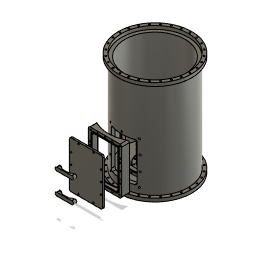
Smooth.SAQ.Pix.Vessel.5.10.2023. (Autodesk Fusion 360 design; units mm, degrees)
Autodesk Fusion 360 part; units mm, degrees
note: some values were not read from the file. Chosen so that the rebuilt part matches the saved one: which bodies a step acts on; which face or edge a step refers to. Set by a fixed rule: which sketch regions a step uses.
(part 1 of 2)
sketch "Vessel.Base" plane through (0, 0, 0) normal (0, 1, 0) x (1, 0, 0)
  circle A0 centre (0, 0) radius 40
  circle A1 centre (0, 0) radius 30
  circle A2 centre (0, 0) radius 100
  circle A3 centre (0, 0) radius 110
  line L0 (0, 0) -> (105, 0) construction
  circle A4 centre (105, 0) radius 2.3
  circle A5 centre (102.3674, 23.3647) radius 2.3
  circle A6 centre (94.6017, 45.5578) radius 2.3
  circle A7 centre (82.0923, 65.4664) radius 2.3
  circle A8 centre (65.4664, 82.0923) radius 2.3
  circle A9 centre (45.5578, 94.6017) radius 2.3
  circle A10 centre (23.3647, 102.3674) radius 2.3
  circle A11 centre (0, 105) radius 2.3
  circle A12 centre (-23.3647, 102.3674) radius 2.3
  circle A13 centre (-45.5578, 94.6017) radius 2.3
  circle A14 centre (-65.4664, 82.0923) radius 2.3
  circle A15 centre (-82.0923, 65.4664) radius 2.3
  circle A16 centre (-94.6017, 45.5578) radius 2.3
  circle A17 centre (-102.3674, 23.3647) radius 2.3
  circle A18 centre (-105, 0) radius 2.3
  circle A19 centre (-102.3674, -23.3647) radius 2.3
  circle A20 centre (-94.6017, -45.5578) radius 2.3
  circle A21 centre (-82.0923, -65.4664) radius 2.3
  circle A22 centre (-65.4664, -82.0923) radius 2.3
  circle A23 centre (-45.5578, -94.6017) radius 2.3
  circle A24 centre (-23.3647, -102.3674) radius 2.3
  circle A25 centre (0, -105) radius 2.3
  circle A26 centre (23.3647, -102.3674) radius 2.3
  circle A27 centre (45.5578, -94.6017) radius 2.3
  circle A28 centre (65.4664, -82.0923) radius 2.3
  circle A29 centre (82.0923, -65.4664) radius 2.3
  circle A30 centre (94.6017, -45.5578) radius 2.3
  circle A31 centre (102.3674, -23.3647) radius 2.3
  circle A32 centre (0, 0) radius 90
  circle A33 centre (0, 0) radius 50
  line L1 (0, 0) -> (45, 0) construction
  circle A34 centre (45, 0) radius 2.3
  circle A35 centre (40.5436, 19.5248) radius 2.3
  circle A36 centre (28.057, 35.1824) radius 2.3
  circle A37 centre (10.0134, 43.8718) radius 2.3
  circle A38 centre (-10.0134, 43.8718) radius 2.3
  circle A39 centre (-28.057, 35.1824) radius 2.3
  circle A40 centre (-40.5436, 19.5248) radius 2.3
  circle A41 centre (-45, 0) radius 2.3
  circle A42 centre (-40.5436, -19.5248) radius 2.3
  circle A43 centre (-28.057, -35.1824) radius 2.3
  circle A44 centre (-10.0134, -43.8718) radius 2.3
  circle A45 centre (10.0134, -43.8718) radius 2.3
  circle A46 centre (28.057, -35.1824) radius 2.3
  circle A47 centre (40.5436, -19.5248) radius 2.3
  circle A48 centre (0, 0) radius 35
  line L2 (0, 0) -> (0, -105) construction
  line L3 (0, 0) -> (0, -95) construction
  circle A49 centre (0, 0) radius 39
  circle A50 centre (0, 0) radius 49
  circle A51 centre (0, 0) radius 48
  circle A52 centre (0, 0) radius 32
  circle A53 centre (0, 0) radius 36 construction
  circle A54 centre (0, 0) radius 37
  circle A55 centre (0, 0) radius 38
  dimension "d1" = 80
  dimension "d2" = 60
  dimension "d3" = 200
  dimension "d4" = 220
  dimension "d5" = 4.6
  dimension "d7" = 360
  dimension "d10" = 180
  dimension "d85" = 100
  dimension "d105" = 45
  dimension "d106" = 4.6
  dimension "d108" = 360
  dimension "d111" = 70
  dimension "d187" = 105
  dimension "d188" = 95
  dimension "d324" = 78
  dimension "d325" = 98
  dimension "d326" = 96
  dimension "d349" = 64
  dimension "d524" = 72
  dimension "d525" = 74
  dimension "d526" = 76
  constraint coincident A0.centre A1.centre
  constraint concentric A1 A2
  constraint concentric A2 A3
  constraint horizontal L0
  constraint coincident L0.end A4.centre
  constraint concentric A0 A33
  constraint horizontal L1
  constraint coincident L1.end A34.centre
  constraint concentric A33 A48
  constraint vertical L2
  constraint parallel L2 L3
  constraint concentric A0 A50
  constraint concentric A48 A52
  constraint concentric A50 A53
  constraint concentric A33 A54
  constraint concentric A0 A55
  measures "d1" diameter of A0
  measures "d2" diameter of A1
  measures "d3" diameter of A2
  measures "d4" diameter of A3
  measures "d5" diameter of A4
  measures "d10" diameter of A32
  measures "d85" diameter of A33
  measures "d105" distance of A0.centre L1.end
  measures "d106" diameter of A34
  measures "d111" diameter of A48
  measures "d187" distance of A0.centre A25.centre
  measures "d188" distance of A0.centre L3.end
  measures "d324" diameter of A49
  measures "d325" diameter of A50
  measures "d326" diameter of A51
  measures "d349" diameter of A52
  measures "d524" diameter of A53
  measures "d525" diameter of A54
  measures "d526" diameter of A55
extrude "Extrude1" add sketch "Vessel.Base" along normal blind 10 contours A3 makes body 1
extrude "Extrude2" add sketch "Vessel.Base" along normal blind 300 separate body contours A2 makes body 2
extrude "Extrude3" add 1 faces at (-98.8073, 10, -35.1548) along direction (0, 1, 0) blind 10 separate body on bodies 1 makes body 3
move_body "Move1" bodies 3 to x (1, 0, 0) y (0, 1, 0) z (0, 0, 1) at (0, 280, 0)
extrude "Extrude5" add sketch "Vessel.Base" along normal blind 10 separate body contours A0 | A48 | A49 | A52 | A54 | A55 makes body 4
extrude "Extrude6" add sketch "Vessel.Base" along normal blind 11.6 contours A32 | A33 | A34 | A35 | A36 | A37 | A38 | A39 | A40 | A41 | A42 | A43 | A44 | A45 | A46 | A47 | A50 | A51 bodies 4
extrude "Extrude7" cut 1 faces at (36.4061, 10, 3.4777) along direction (0, -1, 0) blind 1.6 on bodies 4 bodies 4
sketch "Readout-Holder" plane through (0, 0, 0) normal (0, 1, 0) x (1, 0, 0)
  circle A0 centre (200, 0) radius 30
  circle A1 centre (200, 0) radius 1 construction
  circle A2 centre (210, 0) radius 1 construction
  circle A3 centre (220, 0) radius 1 construction
  circle A4 centre (180, 0) radius 1 construction
  circle A5 centre (205, 8.6603) radius 1 construction
  circle A6 centre (195, 8.6603) radius 1 construction
  circle A7 centre (190, 0) radius 1 construction
  circle A8 centre (195, -8.6603) radius 1 construction
  circle A9 centre (205, -8.6603) radius 1 construction
  circle A10 centre (210, 17.3205) radius 1 construction
  circle A11 centre (190, 17.3205) radius 1 construction
  circle A12 centre (180, 0) radius 1 construction
  circle A13 centre (190, -17.3205) radius 1 construction
  circle A14 centre (210, -17.3205) radius 1 construction
  circle A15 centre (200, 17.3205) radius 1 construction
  circle A16 centre (200, -17.3205) radius 1 construction
  circle A17 centre (185, 8.6603) radius 1 construction
  circle A18 centre (215, 8.6603) radius 1 construction
  circle A19 centre (185, -8.6603) radius 1 construction
  circle A20 centre (215, -8.6603) radius 1 construction
  circle A21 centre (200, 0) radius 40
  circle A22 centre (200, 0) radius 4.5
  circle A23 centre (210, 0) radius 4.5
  circle A24 centre (220, 0) radius 4.5
  circle A25 centre (215, 8.6603) radius 4.5
  circle A26 centre (205, 8.6603) radius 4.5
  circle A27 centre (195, 8.6603) radius 4.5
  circle A28 centre (185, 8.6603) radius 4.5
  circle A29 centre (190, 17.3205) radius 4.5
  circle A30 centre (200, 17.3205) radius 4.5
  circle A31 centre (210, 17.3205) radius 4.5
  circle A32 centre (190, 0) radius 4.5
  circle A33 centre (180, 0) radius 4.5
  circle A34 centre (185, -8.6603) radius 4.5
  circle A35 centre (195, -8.6603) radius 4.5
  circle A36 centre (205, -8.6603) radius 4.5
  circle A37 centre (215, -8.6603) radius 4.5
  circle A38 centre (190, -17.3205) radius 4.5
  circle A39 centre (200, -17.3205) radius 4.5
  circle A40 centre (210, -17.3205) radius 4.5
  circle A41 centre (200, 0) radius 50
  line L0 (200, 0) -> (245, 0) construction
  circle A42 centre (245, 0) radius 2.3
  circle A43 centre (240.5436, 19.5248) radius 2.3
  circle A44 centre (228.057, 35.1824) radius 2.3
  circle A45 centre (210.0134, 43.8718) radius 2.3
  circle A46 centre (189.9866, 43.8718) radius 2.3
  circle A47 centre (171.943, 35.1824) radius 2.3
  circle A48 centre (159.4564, 19.5248) radius 2.3
  circle A49 centre (159.4564, -19.5248) radius 2.3
  circle A50 centre (171.943, -35.1824) radius 2.3
  circle A51 centre (189.9866, -43.8718) radius 2.3
  circle A52 centre (210.0134, -43.8718) radius 2.3
  circle A53 centre (228.057, -35.1824) radius 2.3
  circle A54 centre (240.5436, -19.5248) radius 2.3
  line L1 (215, 8.6603) -> (225, 8.6603) construction
  circle A55 centre (225, 8.6603) radius 1 construction
  circle A56 centre (225, 8.6603) radius 4.5
  circle A57 centre (200, 0) radius 35 construction
  circle A58 centre (200, 0) radius 36.25
  circle A59 centre (200, 0) radius 38.75
  circle A60 centre (200, 0) radius 49
  circle A61 centre (200, 0) radius 34
  circle A62 centre (200, 0) radius 32 construction
  circle A63 centre (200, 0) radius 33
  line L2 (195, -8.6603) -> (185, -8.6603) construction
  line L3 (200, 0) -> (155, 0) construction
  circle A64 centre (155, 0) radius 2.3
  arc A65 (159.4515, 19.5147) -> (155, 0) centre (200, 0) ccw construction
  line L4 (200, 0) -> (159.4515, 19.5147) construction
  line L5 (200, 0) -> (155, 0) construction
  circle A66 centre (200, 0) radius 42
  line L6 (200, 0) -> (200, 35) construction
  circle A67 centre (200, 35) radius 3
  circle A68 centre (169.6891, -17.5) radius 3
  circle A69 centre (230.3109, -17.5) radius 3
  circle A70 centre (200, 32) radius 1
  line L7 (200, 0) -> (200, 32) construction
  circle A71 centre (172.2872, -16) radius 1
  circle A72 centre (227.7128, -16) radius 1
  dimension "d23" = 60
  dimension "d28" = 20
  dimension "d29" = 0
  dimension "d32" = -20
  dimension "d33" = 0
  dimension "d35" = 360
  dimension "d37" = 360
  dimension "d52" = 80
  dimension "d74" = 9
  dimension "d102" = 360
  dimension "d226" = 70
  dimension "d227" = 72.5
  dimension "d228" = 77.5
  dimension "d330" = 98
  dimension "d358" = 68
  dimension "d359" = 64
  dimension "d360" = 66
  dimension "d362" = 10
  dimension "d363" = 45
  dimension "d364" = 4.6
  dimension "d365" = 25.7
  dimension "d378" = 84
  dimension "d397" = 35
  dimension "d398" = 6
  dimension "d400" = 360
  dimension "d404" = 2
  dimension "d405" = 32
  dimension "d407" = 360
  constraint concentric A0 A1
  constraint concentric A0 A21
  constraint concentric A1 A22
  constraint concentric A2 A23
  constraint concentric A3 A24
  constraint concentric A18 A25
  constraint concentric A5 A26
  constraint concentric A6 A27
  constraint concentric A17 A28
  constraint concentric A11 A29
  constraint concentric A15 A30
  constraint concentric A10 A31
  constraint concentric A7 A32
  constraint concentric A12 A33
  constraint concentric A19 A34
  constraint concentric A8 A35
  constraint concentric A9 A36
  constraint concentric A20 A37
  constraint concentric A13 A38
  constraint concentric A16 A39
  constraint concentric A14 A40
  constraint concentric A22 A41
  constraint coincident A0.centre A1.centre
  constraint horizontal L0
  constraint coincident L0.end A42.centre
  constraint horizontal L1
  constraint coincident A18.centre A25.centre
  constraint coincident L1.end A55.centre
  constraint concentric A55 A56
  constraint concentric A41 A57
  constraint concentric A57 A58
  constraint concentric A58 A59
  constraint concentric A1 A60
  constraint concentric A0 A61
  constraint concentric A41 A62
  constraint concentric A0 A63
  constraint coincident A8.centre A35.centre
  constraint horizontal L2
  constraint horizontal L3
  constraint coincident L3.end A64.centre
  constraint concentric A21 A66
  constraint vertical L6
  constraint coincident L6.end A67.centre
  constraint coincident A67 A70.centre
  constraint coincident A62 A70.centre
  constraint parallel L6 L7
  measures "d23" diameter of A0
  measures "d52" diameter of A21
  measures "d74" diameter of A34
  measures "d226" diameter of A57
  measures "d227" diameter of A58
  measures "d228" diameter of A59
  measures "d330" diameter of A60
  measures "d358" diameter of A61
  measures "d359" diameter of A62
  measures "d360" diameter of A63
  measures "d362" distance of A8.centre A19.centre
  measures "d363" distance of A0.centre L3.end
  measures "d364" diameter of A64
  measures "d365" angle of L4 L5
  measures "d378" diameter of A66
  measures "d397" distance of A0.centre L6.end
  measures "d398" diameter of A67
  measures "d404" diameter of A70
  measures "d405" distance of A0.centre A70.centre
extrude "Extrude16" cut sketch "Vessel.Base" along normal blind 18 contours A1 bodies 4
extrude "Extrude17" cut sketch "Vessel.Base" along normal blind 14 contours A0 | A33 | A34 | A35 | A36 | A37 | A38 | A39 | A40 | A41 | A42 | A43 | A44 | A45 | A46 | A47 | A48 | A49 | A50 | A51 | A52 | A54 | A55 bodies 4
extrude "Extrude18" add sketch "Vessel.Base" along normal blind 2 contours A0 | A33 | A34 | A35 | A36 | A37 | A38 | A39 | A40 | A41 | A42 | A43 | A44 | A45 | A46 | A47 | A48 | A49 | A50 | A51 | A52 | A54 | A55 bodies 4
extrude "Extrude19" add 1 faces at (43.0355, 2, 3.9745) along direction (0, 1, 0) blind 4 on bodies 4 bodies 4
extrude "Extrude20" add sketch "Readout-Holder" along normal blind 8 separate body contours A0 A56 | A21 | A41 | A42 | A43 | A44 | A45 | A46 | A47 | A48 | A49 | A50 | A51 | A52 | A53 | A54 | A58 A61 A67 A69 | A58 A61 A67 | A58 A67 | A58 A69 | A58 A61 A69 | A58 A61 A67 A68 | A58 A61 A68 A69 | A61 A63 A67 A69 | A61 A63 A69 | A58 A61 A68 | A58 A68 | A61 A63 A67 A68 | A61 A63 A67 | A61 A63 A68 A69 | A63 A67 A68 A69 A70 A71 A72 | A63 A69 A72 | A61 A63 A68 | A63 A67 A70 | A63 A67 A70 | A63 A69 A72 | A69 A72 | A69 A72 | A63 A68 A71 | A67 A70 | A67 A70 | A63 A68 A71 | A68 A71 | A68 A71 | A59 | A60 | A64 | A66 picked at (228.6545, 9.8725) makes body 5
extrude "Extrude21" cut sketch "Readout-Holder" along normal blind 4 contours A0 A56 | A21 | A41 | A42 | A43 | A44 | A45 | A46 | A47 | A48 | A49 | A50 | A51 | A52 | A53 | A54 | A58 A61 A67 A69 | A58 A61 A67 | A58 A67 | A58 A69 | A58 A61 A69 | A58 A61 A67 A68 | A58 A61 A68 A69 | A61 A63 A67 A69 | A61 A63 A69 | A58 A61 A68 | A58 A68 | A61 A63 A67 A68 | A61 A63 A67 | A61 A63 A68 A69 | A63 A67 A68 A69 A70 A71 A72 | A63 A69 A72 | A61 A63 A68 | A63 A67 A70 | A63 A67 A70 | A63 A69 A72 | A69 A72 | A69 A72 | A63 A68 A71 | A67 A70 | A67 A70 | A63 A68 A71 | A68 A71 | A68 A71 | A59 | A60 | A64 | A66 picked at (228.6545, 9.8725) bodies 5
extrude "Extrude22" add sketch "Readout-Holder" along normal blind 8 contours A0 A56 | A0 A56 picked at (176.7568, 7.7937) picked at (225.7718, 9.0442) bodies 5
extrude "Extrude23" cut sketch "Readout-Holder" along normal blind 20 contours A42 | A43 | A44 | A45 | A46 | A47 | A48 | A49 | A50 | A51 | A52 | A53 | A54 bodies 5
extrude "Extrude24" cut sketch "Vessel.Base" along normal blind 24 contours A34 | A35 | A36 | A37 | A38 | A39 | A40 | A41 | A42 | A43 | A44 | A45 | A46 | A47 bodies 4
extrude "Extrude25" cut sketch "Vessel.Base" along normal blind 1 from surface at 5 contours A0 | A49 | A54 | A55 bodies 4
sketch "Door.Hole" plane through (0, 0, 0) normal (0, 0, 1) x (1, 0, 0)
  line L0 (-35, 30) -> (35, 30)
  line L1 (40, 35) -> (40, 145)
  line L2 (35, 150) -> (-35, 150)
  line L3 (-40, 145) -> (-40, 35)
  line L4 (-45, 20) -> (45, 20)
  line L5 (50, 25) -> (50, 155)
  line L6 (45, 160) -> (-45, 160)
  line L7 (-50, 155) -> (-50, 25)
  circle A0 centre (0, 155) radius 2.3
  circle A1 centre (45, 155) radius 2.3 construction
  circle A2 centre (-45, 111.6667) radius 2.3
  circle A3 centre (45, 111.6667) radius 2.3
  circle A4 centre (-45, 68.3333) radius 2.3
  circle A5 centre (45, 68.3333) radius 2.3
  circle A6 centre (0, 25) radius 2.3
  arc A7 (-35, 150) -> (-40, 145) centre (-35, 145) ccw
  arc A8 (40, 145) -> (35, 150) centre (35, 145) ccw
  arc A9 (-40, 35) -> (-35, 30) centre (-35, 35) ccw
  arc A10 (35, 30) -> (40, 35) centre (35, 35) ccw
  arc A11 (-45, 160) -> (-50, 155) centre (-45, 155) ccw
  arc A12 (50, 155) -> (45, 160) centre (45, 155) ccw
  arc A13 (45, 20) -> (50, 25) centre (45, 25) ccw
  arc A14 (-50, 25) -> (-45, 20) centre (-45, 25) ccw
  line L8 (-35, 155) -> (35, 155) construction
  line L9 (45, 145) -> (45, 35) construction
  line L10 (35, 25) -> (-35, 25) construction
  line L11 (-45, 35) -> (-45, 145) construction
  arc A15 (-35, 155) -> (-45, 145) centre (-35, 145) ccw construction
  arc A16 (45, 145) -> (35, 155) centre (35, 145) ccw construction
  arc A17 (35, 25) -> (45, 35) centre (35, 35) ccw construction
  arc A18 (-45, 35) -> (-35, 25) centre (-35, 35) ccw construction
  line L12 (-34.5711, 152.0711) -> (34.5711, 152.0711)
  line L13 (42.0711, 144.5711) -> (42.0711, 35.4289)
  line L14 (34.5711, 27.9289) -> (-34.5711, 27.9289)
  line L15 (-42.0711, 35.4289) -> (-42.0711, 144.5711)
  arc A19 (-34.5711, 152.0711) -> (-42.0711, 144.5711) centre (-34.5711, 144.5711) ccw
  arc A20 (42.0711, 144.5711) -> (34.5711, 152.0711) centre (34.5711, 144.5711) ccw
  arc A21 (34.5711, 27.9289) -> (42.0711, 35.4289) centre (34.5711, 35.4289) ccw
  arc A22 (-42.0711, 35.4289) -> (-34.5711, 27.9289) centre (-34.5711, 35.4289) ccw
  line L16 (-33.5355, 148.5355) -> (33.5355, 148.5355)
  line L17 (38.5355, 143.5355) -> (38.5355, 36.4645)
  line L18 (33.5355, 31.4645) -> (-33.5355, 31.4645)
  line L19 (-38.5355, 36.4645) -> (-38.5355, 143.5355)
  arc A23 (-33.5355, 148.5355) -> (-38.5355, 143.5355) centre (-33.5355, 143.5355) ccw
  arc A24 (38.5355, 143.5355) -> (33.5355, 148.5355) centre (33.5355, 143.5355) ccw
  arc A25 (33.5355, 31.4645) -> (38.5355, 36.4645) centre (33.5355, 36.4645) ccw
  arc A26 (-38.5355, 36.4645) -> (-33.5355, 31.4645) centre (-33.5355, 36.4645) ccw
  line L20 (-45, 25) -> (-42.0711, 27.9289) construction
  circle A27 centre (-43.3737, 26.6263) radius 2.3
  line L21 (-45, 155) -> (-39.8744, 149.8744) construction
  line L22 (45, 155) -> (39.8744, 149.8744) construction
  line L23 (45, 25) -> (39.8744, 30.1256) construction
  circle A28 centre (43.3737, 26.6263) radius 2.3
  circle A29 centre (-43.3737, 153.3737) radius 2.3
  circle A30 centre (43.3737, 153.3737) radius 2.3
  circle A31 centre (-45, 155) radius 2.3 construction
  circle A32 centre (-45, 25) radius 2.3 construction
  circle A33 centre (45, 25) radius 2.3 construction
  line L24 (33.5355, 31.4645) -> (33.5355, 32.4645) construction
  line L25 (38.5355, 36.4645) -> (37.5355, 36.4645) construction
  line L26 (37.5355, 36.4645) -> (37.5355, 30.6906) construction
  line L27 (33.5355, 32.4645) -> (39.3094, 32.4645) construction
  line L28 (-33.5355, 148.5355) -> (-33.5355, 147.5355) construction
  line L29 (-38.5355, 143.5355) -> (-37.5355, 143.5355) construction
  line L30 (-37.5355, 143.5355) -> (-37.5355, 149.5355) construction
  line L31 (-33.5355, 147.5355) -> (-39.5355, 147.5355) construction
  line L32 (-33.5355, 147.5355) -> (33.5355, 147.5355)
  line L33 (37.5355, 143.5355) -> (37.5355, 36.4645)
  line L34 (33.5355, 32.4645) -> (-33.5355, 32.4645)
  line L35 (-37.5355, 36.4645) -> (-37.5355, 143.5355)
  arc A34 (-33.5355, 147.5355) -> (-37.5355, 143.5355) centre (-33.5355, 143.5355) ccw
  arc A35 (37.5355, 143.5355) -> (33.5355, 147.5355) centre (33.5355, 143.5355) ccw
  arc A36 (33.5355, 32.4645) -> (37.5355, 36.4645) centre (33.5355, 36.4645) ccw
  arc A37 (-37.5355, 36.4645) -> (-33.5355, 32.4645) centre (-33.5355, 36.4645) ccw
  point P0 (-40, 30)
  point P1 (40, 30)
  point P2 (-40, 150)
  point P3 (-50, 20)
  point P4 (50, 20)
  point P5 (-50, 160)
  dimension "d143" = 80
  dimension "d144" = 120
  dimension "d147" = 100
  dimension "d148" = 140
  dimension "d154" = 5
  dimension "d155" = 5
  dimension "d156" = 5
  dimension "d157" = 5
  dimension "d158" = 5
  dimension "d159" = 5
  dimension "d160" = 5
  dimension "d161" = 5
  dimension "d162" = 10
  dimension "d163" = 10
  dimension "d164" = 10
  dimension "d165" = 10
  dimension "d166" = 7.5
  dimension "d167" = 7.5
  dimension "d168" = 7.5
  dimension "d169" = 7.5
  dimension "d170" = 5
  dimension "d171" = 5
  dimension "d172" = 5
  dimension "d173" = 5
  dimension "d174" = 4.6
  dimension "d175" = 4.6
  dimension "d176" = 4.6
  dimension "d177" = 4.6
  dimension "d178" = 4.6
  dimension "d179" = 4.6
  dimension "d180" = 4.6
  dimension "d243" = 1
  dimension "d244" = 1
  dimension "d245" = 1
  dimension "d246" = 1
  dimension "d247" = 6
  dimension "d248" = 6
  dimension "d249" = 4
  dimension "d250" = 4
  dimension "d251" = 4
  dimension "d252" = 4
  constraint horizontal L0
  constraint vertical L1
  constraint horizontal L2
  constraint vertical L3
  constraint horizontal L4
  constraint vertical L5
  constraint horizontal L6
  constraint vertical L7
  constraint coincident P2 L3
  constraint coincident P2 L2
  constraint tangent L3 A7
  constraint tangent L2 A7
  constraint tangent L2 A8
  constraint tangent L1 A8
  constraint coincident P0 L3
  constraint coincident P0 L0
  constraint tangent L3 A9
  constraint tangent L0 A9
  constraint coincident P1 L0
  constraint coincident P1 L1
  constraint tangent L0 A10
  constraint tangent L1 A10
  constraint coincident P5 L7
  constraint coincident P5 L6
  constraint tangent L7 A11
  constraint tangent L6 A11
  constraint tangent L6 A12
  constraint tangent L5 A12
  constraint coincident P4 L4
  constraint coincident P4 L5
  constraint tangent L4 A13
  constraint tangent L5 A13
  constraint coincident P3 L7
  constraint coincident P3 L4
  constraint tangent L7 A14
  constraint tangent L4 A14
  constraint horizontal L8
  constraint vertical L9
  constraint horizontal L10
  constraint vertical L11
  constraint tangent L11 A15
  constraint tangent L8 A15
  constraint tangent L8 A16
  constraint tangent L9 A16
  constraint tangent L10 A17
  constraint tangent L9 A17
  constraint tangent L10 A18
  constraint tangent L11 A18
  constraint horizontal L12
  constraint vertical L13
  constraint horizontal L14
  constraint vertical L15
  constraint tangent L15 A19
  constraint tangent L12 A19
  constraint tangent L12 A20
  constraint tangent L13 A20
  constraint tangent L14 A21
  constraint tangent L13 A21
  constraint tangent L15 A22
  constraint tangent L14 A22
  constraint horizontal L16
  constraint vertical L17
  constraint horizontal L18
  constraint vertical L19
  constraint tangent L19 A23
  constraint tangent L16 A23
  constraint tangent L16 A24
  constraint tangent L17 A24
  constraint tangent L17 A25
  constraint tangent L18 A25
  constraint tangent L19 A26
  constraint tangent L18 A26
  constraint midpoint A18 L20.end
  constraint coincident L20 A27.centre
  constraint coincident A11.centre L21.start
  constraint midpoint A19 L21.end
  constraint coincident A1.centre A12.centre
  constraint midpoint A20 L22.end
  constraint coincident A13.centre L23.start
  constraint midpoint A21 L23.end
  constraint coincident L23 A28.centre
  constraint coincident L21 A29.centre
  constraint coincident A1 A30.centre
  constraint coincident L22 A30.centre
  constraint concentric A11 A31
  constraint coincident A14.centre L20.start
  constraint perpendicular L18 L24
  constraint perpendicular L17 L25
  constraint coincident A10 L26.end
  constraint perpendicular L25 L26
  constraint coincident A10 L27.end
  constraint perpendicular L26 L27
  constraint perpendicular L16 L28
  constraint perpendicular L19 L29
  constraint perpendicular L29 L30
  constraint perpendicular L30 L31
  constraint horizontal L32
  constraint vertical L33
  constraint horizontal L34
  constraint vertical L35
  constraint tangent L35 A34
  constraint tangent L32 A34
  constraint tangent L32 A35
  constraint tangent L33 A35
  constraint tangent L34 A36
  constraint tangent L33 A36
  constraint tangent L34 A37
  constraint tangent L35 A37
  measures "d143" distance of P0 P1
  measures "d144" distance of P0 P2
  measures "d147" distance of P3 P4
  measures "d148" distance of P3 P5
  measures "d154" radius of A7
  measures "d155" radius of A8
  measures "d156" radius of A9
  measures "d157" radius of A10
  measures "d158" radius of A11
  measures "d159" radius of A12
  measures "d160" radius of A13
  measures "d161" radius of A14
  measures "d162" radius of A15
  measures "d163" radius of A16
  measures "d164" radius of A17
  measures "d165" radius of A18
  measures "d166" radius of A19
  measures "d167" radius of A20
  measures "d168" radius of A21
  measures "d169" radius of A22
  measures "d170" radius of A23
  measures "d171" radius of A24
  measures "d172" radius of A25
  measures "d173" radius of A26
  measures "d174" diameter of A27
  measures "d175" diameter of A28
  measures "d176" diameter of A29
  measures "d177" diameter of A30
  measures "d178" diameter of A31
  measures "d179" diameter of A32
  measures "d180" diameter of A33
  measures "d243" distance of L18.start L24.end
  measures "d244" distance of L17.end L25.end
  measures "d245" distance of L16.start L28.end
  measures "d246" distance of L19.end L29.end
  measures "d247" distance of L29.end L30.end
  measures "d248" distance of L28.end L31.end
  measures "d249" radius of A34
  measures "d250" radius of A35
  measures "d251" radius of A36
  measures "d252" radius of A37
extrude "Extrude26" cut sketch "Readout-Holder" along normal blind 9 contours A0 A56 | A0 A56 picked at (225.7718, 9.0442) picked at (228.6545, 9.8725) bodies 5
extrude "Extrude28" add 1 faces at (172.0133, 8, -21.645) along direction (0, 1, 0) blind 6 on bodies 5 bodies 5
extrude "Extrude29" cut 1 faces at (160.1236, 4, 9.3336) along direction (0, 1, 0) blind 2 on bodies 5 bodies 5
extrude "Extrude30" cut 1 faces at (172.0133, 14, -21.645) along direction (0, -1, 0) blind 2 on bodies 5 bodies 5
extrude "Extrude31" cut 1 faces at (172.0133, 12, -21.645) along direction (0, -1, 0) blind 2 on bodies 5 bodies 5
extrude "Extrude35" add sketch "Door.Hole" along normal blind 10 and the other way blind 25 from surface at 95 separate body contours L0 L1 L2 L3 A7 A8 A9 A10 | L4 L5 L6 L7 A11 A12 A13 A14 makes body 6 at (-40, 108.3333, 93.3333) makes body 7 at (-50, 111.6667, 81.6667)
extrude "Extrude36" cut sketch "Vessel.Base" along normal blind 180 contours A2 bodies 6 7 makes body 9 at (-29.4946, 25.286, 95.5514) makes body 8 at (-40, 108.3333, 96.101)
extrude "Extrude37" cut sketch "Door.Hole" along normal blind 180 contours L16 L17 L18 L19 A23 A24 A25 A26 | L32 L33 L34 L35 A34 A35 A36 A37 bodies 2
sketch "Inner.Door.Cleaner" plane through (0, 0, 0) normal (0, 1, 0) x (1, 0, 0)
  circle A0 centre (0, 0) radius 85 construction
  line L0 (0, 0) -> (0, -80) construction
  line L1 (0, -80) -> (25, -80) construction
  line L2 (25, -80) -> (25, -70) construction
  line L3 (25, -70) -> (0, -70) construction
  line L4 (0, -70) -> (0, -80) construction
  line L5 (25, -70) -> (-25, -70)
  line L6 (-25, -70) -> (-25, -70)
  line L7 (-15, -80) -> (15, -80)
  line L8 (25, -70) -> (25, -70)
  arc A1 (-25, -70) -> (-15, -80) centre (-15, -70) ccw
  arc A2 (15, -80) -> (25, -70) centre (15, -70) ccw
  point P0 (14.7189, -80)
  dimension "d198" = 170
  dimension "d199" = 80
  dimension "d200" = 25
  dimension "d201" = 10
  dimension "d202" = 50
  dimension "d203" = 10
  dimension "d204" = 10
  dimension "d205" = 10
  constraint coincident A0.centre L0.start
  constraint vertical L0
  constraint horizontal L1
  constraint vertical L2
  constraint horizontal L3
  constraint vertical L4
  constraint horizontal L5
  constraint horizontal L7
  constraint tangent L7 A1
  constraint coincident P0 L8
  constraint coincident P0 L7
  constraint tangent L7 A2
  measures "d198" diameter of A0
  measures "d199" distance of A0.centre L0.end
  measures "d200" distance of L0.end L1.end
  measures "d201" distance of L0.end L3.end
  measures "d202" distance of L2.end L5.end
  measures "d203" distance of L2.end P0
  measures "d204" radius of A1
  measures "d205" radius of A2
extrude "Extrude38" cut sketch "Inner.Door.Cleaner" along normal blind 175 bodies 6 7
extrude "Extrude39" cut sketch "Door.Hole" along normal blind 130 contours A0 | A2 | A3 | A4 | A5 | A6 | A27 | A28 | A29 | A30 bodies 2
extrude "Extrude40" add sketch "Door.Hole" along normal blind 35 from surface at 70 separate body contours L12 L13 L14 L15 A19 A20 A21 A22 makes body 10
extrude "Extrude41" cut sketch "Vessel.Base" along normal blind 180 contours A2 bodies 10 makes body 11 at (-42.0711, 71.8096, 95.4797)
sketch "Dip.Maker" plane through (0, 0, 0) normal (0, 1, 0) x (1, 0, 0)
  circle A0 centre (0, 0) radius 100
  circle A1 centre (0, 0) radius 101
  circle A2 centre (0, 0) radius 90
  circle A3 centre (0, 0) radius 89
  dimension "d216" = 200
  dimension "d217" = 202
  dimension "d218" = 180
  dimension "d219" = 178
  constraint coincident A0.centre A1.centre
  constraint concentric A0 A1
  constraint concentric A1 A2
  constraint concentric A2 A3
  measures "d216" diameter of A0
  measures "d217" diameter of A1
  measures "d218" diameter of A2
  measures "d219" diameter of A3
extrude "Extrude42" cut sketch "Dip.Maker" along normal blind 155 bodies 10 11
move_body "Move3" bodies 9 to x (1, 0, 0) y (0, 1, 0) z (0, 0, 1) at (0, 0, 60)
move_body "Move4" bodies 8 to x (1, 0, 0) y (0, 1, 0) z (0, 0, 1) at (0, 0, 60)
move_body "Move5" bodies 11 to x (1, 0, 0) y (0, 1, 0) z (0, 0, 1) at (0, 0, 61)
move_body "Move6" bodies 8 9 11 to x (1, 0, 0) y (0, 1, 0) z (0, 0, 1) at (0, 0, 170)
move_body "Move7" bodies 6 to x (1, 0, 0) y (0, 1, 0) z (0, 0, 1) at (0, 0, 110)
move_body "Move8" bodies 7 to x (1, 0, 0) y (0, 1, 0) z (0, 0, 1) at (0, 0, 111)
move_body "Move9" bodies 10 to x (1, 0, 0) y (0, 1, 0) z (0, 0, 1) at (0, 0, 111)
move_body "Move10" bodies 6 to x (1, 0, 0) y (0, 1, 0) z (0, 0, 1) at (0, 0, 1)
sketch "Cleaner.Waste" plane through (0, 160, 0) normal (0, 1, 0) x (-1, 0, 0)
  arc A0 (45, 319.3029) -> (-45, 319.3029) centre (0, 230) ccw
  line L0 (45, 319.3029) -> (45, 335)
  line L1 (45, 335) -> (-45, 335)
  line L2 (-45, 335) -> (-45, 319.3029)
  line L3 (45, 335) -> (-45.0178, 335)
  line L4 (-45.0178, 335) -> (-45.0178, 339.3769)
  line L5 (-45.0178, 339.3769) -> (45, 339.3769)
  line L6 (45, 339.3769) -> (45, 335)
  constraint horizontal L3
  constraint vertical L4
  constraint horizontal L5
  constraint vertical L6
  constraint coincident L0.end L1.start
extrude "Extrude43" cut sketch "Cleaner.Waste" against normal blind 147 contours L1 L3 L4 L5 L6 bodies 11
combine "Combine1" operation add target body 9 tool bodies 11 8
combine "Combine2" operation add target body 7 tool bodies 10 6
move_body "Move11" bodies 7 to x (1, 0, 0) y (0, 1, 0) z (0, 0, 1) at (0, 0, -110)
move_body "Move12" bodies 7 to x (1, 0, 0) y (0, 1, 0) z (0, 0, 1) at (0, 0, -1)
move_body "Move13" bodies 9 to x (1, 0, 0) y (0, 1, 0) z (0, 0, 1) at (0, 0, -220)
move_body "Move14" bodies 9 to x (1, 0, 0) y (0, 1, 0) z (0, 0, 1) at (0, 0, -10)
extrude "Extrude44" add sketch "Readout-Holder" against normal blind 1 from surface at 6 contours A58 A67 | A58 A69 | A58 A68 | A59 bodies 5
extrude "Extrude45" cut 1 faces at (-5, 152.0711, 73.3333) along direction (0, -1, 0) blind 125 on bodies 7 bodies 7
extrude "Extrude46" cut sketch "Door.Hole" against normal blind 1 from surface at 105 contours L12 L13 L14 L15 A19 A20 A21 A22 bodies 9
extrude "Extrude47" add sketch "Door.Hole" against normal blind 5 separate body contours L16 L17 L18 L19 A23 A24 A25 A26 | L32 L33 L34 L35 A34 A35 A36 A37 makes body 12
extrude "Extrude48" add sketch "Door.Hole" along normal blind 5 contours L0 L1 L2 L3 A7 A8 A9 A10 | L12 L13 L14 L15 A19 A20 A21 A22 | L16 L17 L18 L19 A23 A24 A25 A26 | L32 L33 L34 L35 A34 A35 A36 A37 bodies 12
extrude "Extrude49" add sketch "Door.Hole" along normal blind 5 contours L4 L5 L6 L7 A11 A12 A13 A14 | A0 | A2 | A3 | A4 | A5 | A6 | A27 | A28 | A29 | A30 bodies 12
move_body "Move15" bodies 12 to x (1, 0, 0) y (0, 1, 0) z (0, 0, 1) at (0, 0, 120)
move_body "Move16" bodies 12 to x (1, 0, 0) y (0, 1, 0) z (0, 0, 1) at (0, 0, -13)
move_body "Move17" bodies 12 to x (1, 0, 0) y (0, 1, 0) z (0, 0, 1) at (0, 0, 20)
extrude "Extrude50" cut sketch "Door.Hole" against normal blind 1 from surface at 124 contours L16 L17 L18 L19 A23 A24 A25 A26 bodies 12
extrude "Extrude51" cut sketch "Door.Hole" against normal blind 1 from surface at 126 contours L16 L17 L18 L19 A23 A24 A25 A26 bodies 12
extrude "Extrude52" add 2 faces at (-27.0017, 23.7102, 105) (-39.5118, 72.1548, 105) along direction (0, 0, 1) blind 5 on bodies 9 bodies 9
extrude "Extrude53" add 1 faces at (-40.6904, 71.8096, 104) along direction (0, 0, 1) blind 5 on bodies 9 bodies 9
move_body "Move18" bodies 1 to x (1, 0, 0) y (0, 1, 0) z (0, 0, 1) at (0, -20, 0)
move_body "Move19" bodies 3 to x (1, 0, 0) y (0, 1, 0) z (0, 0, 1) at (0, 30, 0)
move_body "Move20" bodies 12 to x (1, 0, 0) y (0, 1, 0) z (0, 0, 1) at (0, 0, 140)
move_body "Move21" bodies 9 to x (1, 0, 0) y (0, 1, 0) z (0, 0, 1) at (0, 0, 60)
move_body "Move22" bodies 7 to x (1, 0, 0) y (0, 1, 0) z (0, 0, 1) at (0, 0, -20)
move_body "Move23" bodies 9 to x (1, 0, 0) y (0, 1, 0) z (0, 0, 1) at (0, 0, -20)
move_body "Move24" bodies 12 to x (1, 0, 0) y (0, 1, 0) z (0, 0, 1) at (0, 0, -60)
move_body "Move25" bodies 1 to x (1, 0, 0) y (0, 1, 0) z (0, 0, 1) at (0, -40, 0)
move_body "Move26" bodies 4 to x (1, 0, 0) y (0, 1, 0) z (0, 0, 1) at (0, -30, 0)
sketch "Door.Design" plane through (0, 0, 212) normal (0, 0, 1) x (1, 0, 0)
  arc A0 (-50, 25) -> (-45, 20) centre (-45, 25) ccw
  line L0 (-45, 20) -> (45, 20)
  arc A1 (45, 20) -> (50, 25) centre (45, 25) ccw
  line L1 (50, 25) -> (50, 155)
  arc A2 (50, 155) -> (45, 160) centre (45, 155) ccw
  line L2 (45, 160) -> (-45, 160)
  arc A3 (-45, 160) -> (-50, 155) centre (-45, 155) ccw
  line L3 (-50, 155) -> (-50, 25)
  line L4 (-48.5355, 158.5355) -> (-45, 155) construction
  line L5 (-45, 155) -> (45, 155) construction
  line L6 (45, 155) -> (48.5355, 158.5355) construction
  line L7 (-45, 155) -> (-45, 25) construction
  line L8 (-45, 25) -> (-48.5355, 21.4645) construction
  line L9 (-45, 25) -> (45, 25) construction
  line L10 (45, 25) -> (48.5355, 21.4645) construction
  line L11 (45, 25) -> (45, 155) construction
  line L12 (0, 155) -> (22.5, 155) construction
  circle A4 centre (22.5, 155) radius 2.3
  line L13 (0, 155) -> (-22.5, 155) construction
  circle A5 centre (-22.5, 155) radius 2.3
  line L14 (-45, 155) -> (-45, 90) construction
  circle A6 centre (-45, 90) radius 2.3
  line L15 (45, 155) -> (45, 90) construction
  circle A7 centre (45, 90) radius 2.3
  line L16 (-45, 155) -> (-45, 122.5) construction
  line L17 (45, 155) -> (45, 122.5) construction
  line L18 (-45, 25) -> (-45, 57.5) construction
  line L19 (45, 25) -> (45, 57.5) construction
  circle A8 centre (-45, 57.5) radius 2.3
  circle A9 centre (45, 57.5) radius 2.3
  circle A10 centre (-45, 122.5) radius 2.3
  circle A11 centre (45, 122.5) radius 2.3
  line L20 (0, 25) -> (22.5, 25) construction
  circle A12 centre (22.5, 25) radius 2.3
  line L21 (0, 25) -> (-22.5, 25) construction
  circle A13 centre (-22.5, 25) radius 2.3
  line L22 (-22.5, 155) -> (-22.5, 25) construction
  line L23 (22.5, 155) -> (22.5, 25) construction
  line L24 (-45, 122.5) -> (45, 122.5) construction
  line L25 (-45, 90) -> (45, 90) construction
  line L26 (-45, 57.5) -> (45, 57.5) construction
  circle A14 centre (-22.5, 122.5) radius 5
  line L27 (-22.5, 127.5) -> (-27.5, 127.5) construction
  line L28 (-27.5, 127.5) -> (-27.5, 122.5) construction
  circle A15 centre (22.5, 122.5) radius 5
  line L29 (22.5, 127.5) -> (27.5, 127.5) construction
  line L30 (27.5, 122.5) -> (27.5, 117.5) construction
  circle A16 centre (-22.5, 57.5) radius 5
  circle A17 centre (22.5, 57.5) radius 5
  line L31 (-22.5, 127.5) -> (22.5, 127.5)
  line L32 (22.5, 117.5) -> (-22.5, 117.5)
  line L33 (-22.5, 62.5) -> (-27.5, 62.5) construction
  line L34 (-22.5, 62.5) -> (22.5, 62.5)
  line L35 (27.5, 57.5) -> (27.5, 57.5)
  line L36 (22.5, 52.5) -> (-22.5, 52.5)
  line L37 (-27.5, 57.5) -> (-27.5, 57.5)
  arc A18 (-22.5, 62.5) -> (-27.5, 57.5) centre (-22.5, 57.5) ccw
  arc A19 (-27.5, 57.5) -> (-22.5, 52.5) centre (-22.5, 57.5) ccw
  arc A20 (27.5, 57.5) -> (22.5, 62.5) centre (22.5, 57.5) ccw
  arc A21 (22.5, 52.5) -> (27.5, 57.5) centre (22.5, 57.5) ccw
  arc A22 (-22.5, 127.5) -> (-27.5, 122.5) centre (-22.5, 122.5) ccw
  arc A23 (-27.5, 122.5) -> (-22.5, 117.5) centre (-22.5, 122.5) ccw
  arc A24 (27.5, 122.5) -> (22.5, 127.5) centre (22.5, 122.5) ccw
  arc A25 (22.5, 117.5) -> (27.5, 122.5) centre (22.5, 122.5) ccw
  point P0 (-27.5, 117.5)
  point P1 (27.5, 62.5)
  point P2 (-27.5, 52.5)
  dimension "d263" = 22.5
  dimension "d264" = 4.6
  dimension "d265" = 22.5
  dimension "d266" = 4.6
  dimension "d267" = 65
  dimension "d268" = 4.6
  dimension "d269" = 4.6
  dimension "d270" = 32.5
  dimension "d271" = 32.5
  dimension "d272" = 4.6
  dimension "d273" = 4.6
  dimension "d274" = 4.6
  dimension "d275" = 4.6
  dimension "d276" = 22.5
  dimension "d277" = 4.6
  dimension "d278" = 22.5
  dimension "d279" = 4.6
  dimension "d282" = 10
  dimension "d283" = 5
  dimension "d284" = 10
  dimension "d285" = 10
  dimension "d286" = 5
  dimension "d287" = 10
  dimension "d288" = 10
  dimension "d289" = 10
  dimension "d290" = 5
  dimension "d291" = 55
  dimension "d292" = 10
  dimension "d293" = 5
  dimension "d294" = 5
  dimension "d295" = 5
  dimension "d296" = 5
  dimension "d297" = 5
  dimension "d298" = 5
  dimension "d299" = 5
  dimension "d300" = 5
  constraint midpoint A3 L4.start
  constraint coincident A3.centre L4.end
  constraint coincident A2.centre L5.end
  constraint midpoint A2 L6.end
  constraint coincident A0.centre L7.end
  constraint midpoint A0 L8.end
  constraint coincident A1.centre L9.end
  constraint midpoint A1 L10.end
  constraint midpoint L5 L12.start
  constraint coincident L5 L12.end
  constraint coincident L12.end A4.centre
  constraint coincident L5 L13.end
  constraint coincident L13.end A5.centre
  constraint perpendicular L9 L14
  constraint coincident L14.end A6.centre
  constraint midpoint L11 L15.end
  constraint coincident L15.end A7.centre
  constraint midpoint L14 L16.end
  constraint midpoint L15 L17.end
  constraint perpendicular L9 L18
  constraint perpendicular L9 L19
  constraint coincident L18.end A8.centre
  constraint coincident L19.end A9.centre
  constraint coincident L16.end A10.centre
  constraint coincident L17.end A11.centre
  constraint midpoint L9 L20.start
  constraint parallel L9 L20
  constraint coincident L20.end A12.centre
  constraint parallel L9 L21
  constraint coincident L21.end A13.centre
  constraint coincident L22 A14.centre
  constraint coincident L24 A14.centre
  constraint coincident A14 L27.start
  constraint coincident L22 L27.start
  constraint perpendicular L22 L27
  constraint vertical L28
  constraint coincident L24 A15.centre
  constraint coincident L23 A15.centre
  constraint horizontal L29
  constraint coincident A15 L29.start
  constraint coincident L23 L29.start
  constraint perpendicular L24 L30
  constraint coincident L22 A16.centre
  constraint coincident L26 A16.centre
  constraint coincident L26 A17.centre
  constraint coincident L23 A17.centre
  constraint horizontal L31
  constraint horizontal L32
  constraint horizontal L33
  constraint coincident A16 L33.start
  constraint coincident L22 L33.start
  constraint horizontal L34
  constraint horizontal L36
  constraint coincident L33.end L34
  constraint tangent L34 A18
  constraint coincident P2 L37
  constraint coincident P2 L36
  constraint tangent L36 A19
  constraint coincident P1 L34
  constraint tangent L34 A20
  constraint tangent L36 A21
  constraint coincident L27.end L31
  constraint tangent L31 A22
  constraint coincident P0 L28
  constraint tangent L28 A23
  constraint tangent L32 A23
  constraint coincident L29.end L30
  constraint tangent L31 A24
  constraint tangent L30 A24
  constraint coincident L30.end L32
  constraint tangent L32 A25
  measures "d263" distance of L12.start L12.end
  measures "d264" diameter of A4
  measures "d265" distance of L12.start L13.end
  measures "d266" diameter of A5
  measures "d267" distance of A3.centre L14.end
  measures "d268" diameter of A6
  measures "d269" diameter of A7
  measures "d270" distance of A0.centre L18.end
  measures "d271" distance of A1.centre L19.end
  measures "d272" diameter of A8
  measures "d273" diameter of A9
  measures "d274" diameter of A10
  measures "d275" diameter of A11
  measures "d276" distance of L20.start L20.end
  measures "d277" diameter of A12
  measures "d278" distance of L20.start L21.end
  measures "d279" diameter of A13
  measures "d282" diameter of A14
  measures "d283" distance of L27.start L27.end
  measures "d284" distance of L27.end P0
  measures "d285" diameter of A15
  measures "d286" distance of L29.start L29.end
  measures "d287" distance of L29.end L30.end
  measures "d288" diameter of A16
  measures "d289" diameter of A17
  measures "d290" distance of L33.start L33.end
  measures "d291" distance of L33.end P1
  measures "d292" distance of L33.end P2
  measures "d293" radius of A18
  measures "d294" radius of A19
  measures "d295" radius of A20
  measures "d296" radius of A21
  measures "d297" radius of A22
  measures "d298" radius of A23
  measures "d299" radius of A24
  measures "d300" radius of A25
extrude "Extrude54" cut sketch "Door.Design" against normal blind 72 contours A4 | A5 | A6 | A7 | A8 | A9 | A10 | A11 | A12 | A13 bodies 9 12
extrude "Extrude56" add sketch "Door.Design" along normal blind 8 from surface at 2 separate body contours A14 A22 A23 | A14 A15 L31 L32 | A15 A24 A25 | A16 A18 A19 | A16 A17 L34 L36 | A17 A20 A21 makes body 13 at (7.5, 120.8333, 214) makes body 14 at (7.5, 55.8333, 214)
extrude "Extrude57" add sketch "Door.Design" along normal blind 2 separate body contours A14 A22 A23 | A15 A24 A25 | A16 A18 A19 | A17 A20 A21 makes body 15 at (24.0202, 122.0253, 212) makes body 16 at (-21.0489, 56.0699, 212) makes body 17 at (-20.9798, 122.0253, 212) makes body 18 at (23.9511, 56.0699, 212)
sketch "Door.Handle" plane through (0, 127.5, 0) normal (0, 1, 0) x (-1, 0, 0)
  line L0 (-22.5, 214) -> (22.5, 214)
  line L1 (22.5, 214) -> (22.5, 222)
  line L2 (22.5, 222) -> (-22.5, 222)
  line L3 (-22.5, 222) -> (-22.5, 214)
  line L4 (22.5, 214) -> (22.5, 212) construction
  line L5 (22.5, 212) -> (-22.5, 212) construction
  line L6 (-22.5, 212) -> (-22.5, 222) construction
  line L7 (-22.5, 222) -> (22.5, 222) construction
  line L8 (22.5, 222) -> (22.5, 212) construction
  line L9 (22.5, 214) -> (17.5, 214) construction
  line L10 (17.5, 214) -> (-17.5, 214)
  line L11 (-17.5, 214) -> (-17.5, 209)
  line L12 (-7.5, 219) -> (7.5, 219)
  line L13 (17.5, 209) -> (17.5, 214)
  arc A0 (17.5, 209) -> (7.5, 219) centre (7.5, 209) ccw
  arc A1 (-7.5, 219) -> (-17.5, 209) centre (-7.5, 209) ccw
  point P0 (17.5, 219)
  dimension "d308" = 2
  dimension "d309" = 5
  dimension "d310" = 35
  dimension "d311" = 5
  dimension "d312" = 10
  dimension "d313" = 10
  constraint coincident L0.end L1.start
  constraint perpendicular L0 L4
  constraint horizontal L5
  constraint vertical L6
  constraint horizontal L7
  constraint vertical L8
  constraint coincident L2.end L3.start
  constraint perpendicular L4 L9
  constraint horizontal L10
  constraint vertical L11
  constraint horizontal L12
  constraint vertical L13
  constraint coincident P0 L13
  constraint coincident P0 L12
  constraint tangent L13 A0
  constraint tangent L12 A0
  constraint tangent L12 A1
  constraint tangent L11 A1
  measures "d308" distance of L0.end L4.end
  measures "d309" distance of L0.end L9.end
  measures "d310" distance of L9.end L10.end
  measures "d311" distance of L9.end P0
  measures "d312" radius of A0
  measures "d313" radius of A1
extrude "Extrude58" cut sketch "Door.Handle" against normal blind 91 contours L0 L10 L12 A0 A1 bodies 13 14
move_body "Move27" bodies 12 to x (1, 0, 0) y (0, 1, 0) z (0, 0, 1) at (0, 0, -15)
combine "Combine3" operation add target body 14 tool bodies 18 16
combine "Combine4" operation add target body 13 tool bodies 17 15
move_body "Move28" bodies 3 to x (1, 0, 0) y (0, 1, 0) z (0, 0, 1) at (0, -70, 0)
sketch "Vessel.Top" plane through (0, 300, 0) normal (0, 1, 0) x (-1, 0, 0)
  circle A0 centre (0, 0) radius 90 construction
  circle A1 centre (0, 0) radius 100 construction
  circle A2 centre (0, 0) radius 30 construction
  circle A3 centre (0, 0) radius 40 construction
  dimension "d316" = 60
  dimension "d317" = 80
  constraint coincident A0.centre A1.centre
  constraint concentric A2 A3
  measures "d316" diameter of A2
  measures "d317" diameter of A3
move_body "Move29" bodies 5 to x (1, 0, 0) y (0, 1, 0) z (0, 0, 1) at (-200, 0, 0)
move_body "Move30" bodies 5 to x (1, 0, 0) y (0, 1, 0) z (0, 0, 1) at (0, -30, 0)
move_body "Move31" bodies 5 to x (1, 0, 0) y (0, 1, 0) z (0, 0, 1) at (200, 0, 0)
extrude "Extrude59" add sketch "Readout-Holder" along normal blind 1 separate body contours A58 A67 | A58 A69 | A58 A68 | A59 makes body 19
move_body "Move32" bodies 19 to x (1, 0, 0) y (0, 1, 0) z (0, 0, 1) at (-200, 0, 0)
move_body "Move33" bodies 19 to x (1, 0, 0) y (0, 1, 0) z (0, 0, 1) at (0, -25, 0)
combine "Combine5" operation add target body 4 tool bodies 19
move_body "Move34" bodies 5 to x (1, 0, 0) y (0, 1, 0) z (0, 0, 1) at (0, 24, 0)
extrude "Extrude60" cut 1 faces at (173.6203, -1, -27.103) along direction (0, 1, 0) blind 2 on bodies 5 bodies 5
extrude "Extrude61" add 1 faces at (173.6203, 1, -27.103) along direction (0, -1, 0) blind 1 on bodies 5 bodies 5
move_body "Move35" bodies 4 to x (1, 0, 0) y (0, 1, 0) z (0, 0, 1) at (0, 30, 0)
extrude "Extrude62" cut sketch "Vessel.Base" along normal blind 1 from surface at 5 contours A50 bodies 4
extrude "Extrude63" cut sketch "Readout-Holder" along normal blind 1 from surface at 1 contours A41 bodies 5
extrude "Extrude64" cut sketch "Readout-Holder" along normal blind 1 from surface at 3 contours A41 bodies 5
extrude "Extrude65" add 1 faces at (151.4424, 3, 9.831) along direction (0, 1, 0) blind 1 on bodies 5 bodies 5
extrude "Extrude66" add 1 faces at (172.0133, 4, -21.645) along direction (0, 1, 0) blind 2 on bodies 5 bodies 5
extrude "Extrude67" add sketch "Readout-Holder" against normal blind 2 from surface at 6 contours A42 | A43 | A44 | A45 | A46 | A47 | A48 | A49 | A50 | A51 | A52 | A53 | A54 | A60 bodies 5
extrude "Extrude68" cut sketch "Readout-Holder" along normal blind 1 from surface at 4 contours A41 bodies 5
move_body "Move36" bodies 5 to x (1, 0, 0) y (0, 1, 0) z (0, 0, 1) at (-200, 5, 0)
move_body "Move37" bodies 5 to x (1, 0, 0) y (0, 1, 0) z (0, 0, 1) at (0, 1, 0)
move_body "Move38" bodies 5 to x (1, 0, 0) y (0, 1, 0) z (0, 0, 1) at (0, -30, 0)
extrude "Extrude69" add 1 faces at (76.3316, 11.6, 4.4713) along direction (0, 1, 0) blind 2 on bodies 4 bodies 4
move_body "Move39" bodies 5 to x (1, 0, 0) y (0, 1, 0) z (0, 0, 1) at (0, 30, 0)
extrude "Extrude70" cut sketch "Vessel.Base" along normal blind 14 contours A52 bodies 4
move_body "Move40" bodies 5 to x (1, 0, 0) y (0, 1, 0) z (0, 0, 1) at (0, -20, 0)
extrude "Extrude71" add sketch "Vessel.Base" against normal blind 7 from surface at -13 contours A52 bodies 5
move_body "Move41" bodies 5 to x (1, 0, 0) y (0, 1, 0) z (0, 0, 1) at (0, 130, 0)
extrude "Extrude72" cut 1 faces at (28.6545, 117, -9.8725) along direction (0, -1, 0) blind 12 on bodies 5 bodies 5
move_body "Move42" bodies 5 to x (1, 0, 0) y (0, 1, 0) z (0, 0, 1) at (200, 0, 0)
move_body "Move43" bodies 5 to x (1, 0, 0) y (0, 1, 0) z (0, 0, 1) at (0, -110, 0)
extrude "Extrude73" add sketch "Readout-Holder" along normal blind 6.5 contours A61 A63 A67 A69 | A61 A63 A69 | A61 A63 A67 A68 | A61 A63 A67 | A61 A63 A68 A69 | A63 A67 A68 A69 A70 A71 A72 | A63 A69 A72 | A61 A63 A68 | A63 A67 A70 | A63 A67 A70 | A63 A69 A72 | A69 A72 | A69 A72 | A63 A68 A71 | A67 A70 | A67 A70 | A63 A68 A71 | A68 A71 | A68 A71 bodies 5
extrude "Extrude74" cut sketch "Readout-Holder" along normal blind 1 from surface at 1 contours A61 A63 A67 A69 | A61 A63 A69 | A61 A63 A67 A68 | A61 A63 A67 | A61 A63 A68 A69 | A61 A63 A68 bodies 5
extrude "Extrude75" cut sketch "Readout-Holder" along normal blind 1 from surface at 4 contours A61 A63 A67 A69 | A61 A63 A69 | A61 A63 A67 A68 | A61 A63 A67 | A61 A63 A68 A69 | A61 A63 A68 bodies 5
extrude "Extrude76" cut sketch "Readout-Holder" along normal blind 10 contours A64 bodies 5
move_body "Move44" bodies 5 to x (1, 0, 0) y (0, 1, 0) z (0, 0, 1) at (-200, 16, 0)
move_body "Move45" bodies 5 to x (1, 0, 0) y (0, 1, 0) z (0, 0, 1) at (0, 12, 0)
extrude "Extrude77" cut 1 faces at (20.9098, 28, -17.9888) along direction (0, -1, 0) blind 29 on bodies 5 bodies 4
move_body "Move46" bodies 5 to x (1, 0, 0) y (0, 1, 0) z (0, 0, 1) at (0, -28, 0)
move_body "Move47" bodies 5 to x (1, 0, 0) y (0, 1, 0) z (0, 0, 1) at (200, 0, 0)
extrude "Extrude79" add sketch "Readout-Holder" along normal blind 1 from surface at 12 contours A66 bodies 5
move_body "Move48" bodies 5 to x (1, 0, 0) y (0, 1, 0) z (0, 0, 1) at (-200, 0, 0)
move_body "Move49" bodies 5 to x (1, 0, 0) y (0, 1, 0) z (0, 0, 1) at (0, 20, 0)
extrude "Extrude80" add 1 faces at (-16.986, 33, -37.5682) along direction (0, 1, 0) blind 0.6 on bodies 5 bodies 5
extrude "Extrude81" add 1 faces at (46.9908, 32, 4.5706) along direction (0, 1, 0) blind 1.6 on bodies 5 bodies 5
move_body "Move50" bodies 14 13 to x (1, 0, 0) y (0, 1, 0) z (0, 0, 1) at (0, 0, 50)
move_body "Move51" bodies 12 to x (1, 0, 0) y (0, 1, 0) z (0, 0, 1) at (0, 0, 10)